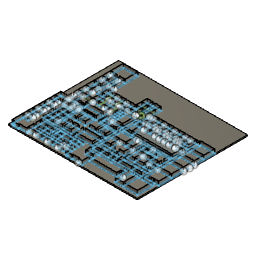
hospital_v5_v1 (Autodesk Fusion 360 design; units mm, degrees)
Autodesk Fusion 360 part; units mm, degrees
(part 1 of 2)
sketch "Sketch1" plane through (0, 0, 0) normal (0, 1, 0) x (1, 0, 0)
  line L0 (-43200, 1200) -> (-48800, 1200)
  line L1 (-48800, 1200) -> (-48800, -38423.7542)
  line L2 (-48800, -38423.7542) -> (-47000, -38423.7542)
  line L3 (-47000, -38423.7542) -> (-47000, -39400)
  line L4 (-47000, -39400) -> (-42700, -39400)
  line L5 (-42700, -39400) -> (-42700, -38500)
  line L6 (-42700, -38500) -> (-36000, -38500)
  line L7 (-36000, -38500) -> (-36000, -37042.096)
  line L8 (-43200, 900) -> (-48500, 900)
  line L9 (-48500, 900) -> (-48500, -38123.7542)
  line L10 (-48500, -38123.7542) -> (-46700, -38123.7542)
  line L11 (-46700, -38123.7542) -> (-46700, -39100)
  line L12 (-46700, -39100) -> (-43000, -39100)
  line L13 (-43000, -39100) -> (-43000, -38200)
  line L14 (-43000, -38200) -> (-36300, -38200)
  line L15 (-36300, -38200) -> (-36300, -37042.096)
  line L16 (-43200, 1200) -> (-43200, 4000)
  line L17 (-43200, 4000) -> (-42900, 4000)
  line L18 (-42900, 4000) -> (-42900, 2400)
  line L19 (-42900, 2400) -> (-39400, 2400)
  line L20 (-39400, 2400) -> (-39400, 9200)
  line L21 (-39400, 9200) -> (-42900, 9200)
  line L22 (-42900, 9200) -> (-42900, 5600)
  line L23 (-42900, 5600) -> (-43200, 5600)
  line L24 (-43200, 5600) -> (-43200, 45841.5562)
  line L25 (-43200, 45841.5562) -> (-31093.7265, 45841.5562)
  line L26 (-31093.7265, 45841.5562) -> (-31093.7265, 22000)
  line L27 (-31093.7265, 22000) -> (-9000, 22000)
  line L28 (-9000, 22000) -> (-9000, 31000)
  line L29 (-9000, 31000) -> (-4200, 31000)
  line L30 (-4200, 31000) -> (-4200, 27800)
  line L31 (-43200, 3700) -> (-43200, 2100)
  line L32 (-43200, 9500) -> (-43200, 5900)
  line L33 (-4500, 30700) -> (-4500, 27800)
  line L34 (-8700, 30700) -> (-4500, 30700)
  line L35 (-31393.7265, 21700) -> (-8700, 21700)
  line L36 (-31393.7265, 45541.5562) -> (-31393.7265, 21700)
  line L37 (-42900, 45541.5562) -> (-31393.7265, 45541.5562)
  line L38 (-42900, 9500) -> (-42900, 45541.5562)
  line L39 (-39100, 9500) -> (-42900, 9500)
  line L40 (-39100, 2100) -> (-39100, 9500)
  line L41 (-42900, 2100) -> (-39100, 2100)
  line L42 (-42900, 900) -> (-42900, 2100)
  line L43 (-42900, 900) -> (-48500, 900)
  line L44 (-48500, 900) -> (-48500, -38123.7542)
  line L45 (-48500, -38123.7542) -> (-46700, -38123.7542)
  line L46 (-46700, -38123.7542) -> (-46700, -39100)
  line L47 (-46700, -39100) -> (-43000, -39100)
  line L48 (-43000, -39100) -> (-43000, -38200)
  line L49 (-43000, -38200) -> (-36300, -38200)
  line L50 (-36300, -38200) -> (-36300, -37042.096)
  line L51 (-4200, 27800) -> (-4500, 27800)
  line L52 (-42900, 35048.3109) -> (-42900, 35074.8344)
  line L53 (-42900, 29017.6863) -> (-38000, 29017.6863)
  line L54 (-38000, 29017.6863) -> (-38000, 34000)
  line L55 (-42900, 35646.5956) -> (-37766.6149, 35646.5956)
  line L56 (-37766.6149, 35646.5956) -> (-37766.6149, 35346.5956)
  line L57 (-37766.6149, 35346.5956) -> (-42900, 35346.5956)
  line L58 (-42900, 35346.5956) -> (-42900, 35646.5956)
  line L59 (-35993.9818, 35346.5956) -> (-31393.7265, 35346.5956)
  line L60 (-31393.7265, 35346.5956) -> (-31393.7265, 35646.5956)
  line L61 (-31393.7265, 35646.5956) -> (-35993.9818, 35646.5956)
  line L62 (-35993.9818, 35646.5956) -> (-35993.9818, 35346.5956)
  line L63 (-42900, 28717.6863) -> (-37700, 28717.6863)
  line L64 (-37700, 28717.6863) -> (-37700, 34000)
  line L65 (-38000, 34000) -> (-37700, 34000)
  line L66 (-37700, 28717.6863) -> (-37700, 23500)
  line L67 (-37700, 23500) -> (-38000, 23500)
  line L68 (-38000, 23500) -> (-38000, 28717.6863)
  line L69 (-38000, 22500) -> (-42900, 22500)
  line L70 (-42900, 22500) -> (-42900, 22200)
  line L71 (-42900, 22200) -> (-38000, 22200)
  line L72 (-38000, 22200) -> (-38000, 22500)
  line L73 (-42900, 15894.4389) -> (-38184.1215, 15894.4389)
  line L74 (-38184.1215, 15894.4389) -> (-38184.1215, 21000)
  line L75 (-38184.1215, 21000) -> (-37884.1215, 21000)
  line L76 (-37884.1215, 21000) -> (-37884.1215, 10500)
  line L77 (-37884.1215, 15594.4389) -> (-37884.1215, 20700)
  line L78 (-42900, 15594.4389) -> (-38184.1215, 15594.4389)
  line L79 (-38184.1215, 15594.4389) -> (-38184.1215, 10500)
  line L80 (-38184.1215, 10500) -> (-37884.1215, 10500)
  line L81 (-31393.7265, 26975.7665) -> (-35176.305, 26975.7665)
  line L82 (-35176.305, 26975.7665) -> (-35176.305, 34204.0089)
  line L83 (-35176.305, 34204.0089) -> (-35476.305, 34204.0089)
  line L84 (-35476.305, 34204.0089) -> (-35476.305, 18232.4873)
  line L85 (-35476.305, 18232.4873) -> (-35176.305, 18232.4873)
  line L86 (-35476.305, 26675.7665) -> (-35476.305, 33904.0089)
  line L87 (-31393.7265, 26675.7665) -> (-35176.305, 26675.7665)
  line L88 (-35176.305, 26675.7665) -> (-35176.305, 18532.4873)
  line L89 (-35176.305, 18232.4873) -> (-35176.305, 18532.4873)
  line L90 (-31393.7265, 21700) -> (-31393.7265, 17176.0979)
  line L91 (-31393.7265, 17176.0979) -> (-35500, 17176.0979)
  line L92 (-35500, 17176.0979) -> (-35500, 16876.0979)
  line L93 (-35500, 16876.0979) -> (-29216.2, 16876.0979)
  line L94 (-29216.2, 16876.0979) -> (-29216.2, 17026.0979)
  line L95 (-29216.2, 17026.0979) -> (-29216.2, 17176.0979)
  line L96 (-29216.2, 17176.0979) -> (-31100, 17176.0979)
  line L97 (-31100, 17176.0979) -> (-31100, 21700)
  line L98 (-27716.2, 16974.86) -> (-28016.2, 16974.86)
  line L99 (-28016.2, 16974.86) -> (-28016.2, 21700)
  line L100 (-28016.2, 21700) -> (-27716.2, 21700)
  line L101 (-27716.2, 21700) -> (-27716.2, 16974.86)
  line L102 (-24100, 21700) -> (-24100, 17200)
  line L103 (-24100, 17200) -> (-26516.2, 17200)
  line L104 (-26516.2, 17200) -> (-26516.2, 16900)
  line L105 (-26516.2, 16900) -> (-21500, 16900)
  line L106 (-23800, 16900) -> (-26216.2, 16900)
  line L107 (-23800, 21700) -> (-23800, 17200)
  line L108 (-23800, 17200) -> (-21500, 17200)
  line L109 (-21500, 16900) -> (-21500, 17200)
  line L110 (-20100, 16900) -> (-20400, 16900)
  line L111 (-20400, 16900) -> (-20400, 21700)
  line L112 (-20400, 21700) -> (-20100, 21700)
  line L113 (-20100, 21700) -> (-20100, 16900)
  line L114 (-16700, 21700) -> (-16700, 17300)
  line L115 (-16700, 17300) -> (-18900, 17300)
  line L116 (-18900, 17300) -> (-18900, 17000)
  line L117 (-18900, 17000) -> (-14100, 17000)
  line L118 (-16400, 17000) -> (-18600, 17000)
  line L119 (-16400, 21700) -> (-16400, 17300)
  line L120 (-16400, 17300) -> (-14100, 17300)
  line L121 (-14100, 17300) -> (-14100, 17000)
  line L122 (-13000, 17000) -> (-12700, 17000)
  line L123 (-12700, 17000) -> (-12700, 21700)
  line L124 (-12700, 21700) -> (-13000, 21700)
  line L125 (-13000, 21700) -> (-13000, 17000)
  line L126 (-8700, 21700) -> (-8700, 17200)
  line L127 (-8700, 17200) -> (-11200, 17200)
  line L128 (-11200, 17200) -> (-11200, 16900)
  line L129 (-11200, 16900) -> (-4300, 16900)
  line L130 (-4300, 16900) -> (-4300, 17200)
  line L131 (-4300, 17200) -> (-8400, 17200)
  line L132 (-4600, 16900) -> (-8400, 16900)
  line L133 (-8400, 16900) -> (-10900, 16900)
  line L134 (-8400, 21700) -> (-8400, 17200)
  line L135 (-8400, 17200) -> (-4600, 17200)
  line L136 (-8400, 21700) -> (-8400, 21900)
  line L137 (-8400, 21900) -> (-4500, 21900)
  line L138 (-4500, 21900) -> (-4500, 18400)
  line L139 (-4500, 18400) -> (-4200, 18400)
  line L140 (-4200, 18400) -> (-4200, 22200)
  line L141 (-4200, 22200) -> (-8684.9202, 22200)
  line L142 (-8684.9202, 22200) -> (-8684.9202, 26300)
  line L143 (-8684.9202, 26300) -> (-4500, 26300)
  line L144 (-4500, 26300) -> (-4500, 23100)
  line L145 (-4500, 23100) -> (-4200, 23100)
  line L146 (-4200, 23100) -> (-4200, 26600)
  line L147 (-4200, 26600) -> (-8400, 26600)
  line L148 (-8700, 30700) -> (-8700, 26600)
  line L149 (-8700, 26600) -> (-8400, 26600)
  line L150 (-2627.1706, 27699.3854) -> (-2627.1706, 30999.3854)
  line L151 (-2627.1706, 30999.3854) -> (2372.8294, 30999.3854)
  line L152 (2372.8294, 30999.3854) -> (2372.8294, 22038.2459)
  line L153 (2372.8294, 22038.2459) -> (42278.3615, 22038.2459)
  line L154 (42278.3615, 22038.2459) -> (42278.3615, 22999.3854)
  line L155 (42278.3615, 22999.3854) -> (53772.8294, 22999.3854)
  line L156 (53772.8294, 22999.3854) -> (53772.8294, 2299.3854)
  line L157 (-2327.1706, 27699.3854) -> (-2327.1706, 30699.3854)
  line L158 (-2327.1706, 30699.3854) -> (2072.8294, 30699.3854)
  line L159 (2072.8294, 30699.3854) -> (2072.8294, 21738.2459)
  line L160 (2072.8294, 21738.2459) -> (42578.3615, 21738.2459)
  line L161 (42578.3615, 21738.2459) -> (42578.3615, 22699.3854)
  line L162 (42578.3615, 22699.3854) -> (53472.8294, 22699.3854)
  line L163 (53472.8294, 22699.3854) -> (53472.8294, 2299.3854)
  line L164 (-2627.1706, 27699.3854) -> (-2327.1706, 27699.3854)
  line L165 (-2600, 22900) -> (-2600, 26500)
  line L166 (-2600, 26500) -> (2072.8294, 26500)
  line L167 (-2600, 22900) -> (-2300, 22900)
  line L168 (-2300, 22900) -> (-2300, 26200)
  line L169 (-2300, 26200) -> (2072.8294, 26200)
  line L170 (-2400, 22200) -> (2072.8294, 22200)
  line L171 (2072.8294, 22200) -> (2072.8294, 21900)
  line L172 (2072.8294, 21900) -> (-2400, 21900)
  line L173 (-2400, 21900) -> (-2400, 22200)
  line L174 (1800, 21900) -> (1800, 19900)
  line L175 (1800, 19900) -> (4200, 19900)
  line L176 (2100, 21900) -> (2100, 20200)
  line L177 (2100, 20200) -> (4200, 20200)
  line L178 (4200, 19900) -> (4200, 20200)
  line L179 (2100, 19500) -> (2100, 17000)
  line L180 (2100, 17000) -> (-2200, 17000)
  line L181 (-2200, 17000) -> (-2200, 19500)
  line L182 (1400, 19500) -> (1400, 17700)
  line L183 (1400, 17700) -> (-1300, 17700)
  line L184 (-1300, 17700) -> (-1300, 19500)
  line L185 (-2200, 19500) -> (-1300, 19500)
  line L186 (1400, 19500) -> (2100, 19500)
  line L187 (5059.5443, 21738.2459) -> (5059.5443, 17199.3854)
  line L188 (5059.5443, 17199.3854) -> (8300, 17199.3854)
  line L189 (5359.5443, 21738.2459) -> (5359.5443, 17499.3854)
  line L190 (5359.5443, 17499.3854) -> (8300, 17499.3854)
  line L191 (8300, 17199.3854) -> (8300, 17499.3854)
  line L192 (9400, 17200) -> (9700, 17200)
  line L193 (9700, 17200) -> (9700, 21738.2459)
  line L194 (9700, 21738.2459) -> (9400, 21738.2459)
  line L195 (9400, 21738.2459) -> (9400, 17200)
  line L196 (13696.8067, 21738.2459) -> (13696.8067, 17599.3854)
  line L197 (13696.8067, 17599.3854) -> (10700, 17599.3854)
  line L198 (10700, 17599.3854) -> (10700, 17299.3854)
  line L199 (10700, 17299.3854) -> (16618.3238, 17299.3854)
  line L200 (13996.8067, 17299.3854) -> (11000, 17299.3854)
  line L201 (13996.8067, 21738.2459) -> (13996.8067, 17599.3854)
  line L202 (13996.8067, 17599.3854) -> (16618.3238, 17599.3854)
  line L203 (16618.3238, 17299.3854) -> (16618.3238, 17599.3854)
  line L204 (18000, 17400) -> (18300, 17400)
  line L205 (18300, 17400) -> (18300, 21738.2459)
  line L206 (18300, 21738.2459) -> (18000, 21738.2459)
  line L207 (18000, 21738.2459) -> (18000, 17400)
  line L208 (22221.7642, 21738.2459) -> (22221.7642, 17599.3854)
  line L209 (22221.7642, 17599.3854) -> (19200, 17599.3854)
  line L210 (19200, 17599.3854) -> (19200, 17299.3854)
  line L211 (19200, 17299.3854) -> (25200, 17299.3854)
  line L212 (22521.7642, 17299.3854) -> (19500, 17299.3854)
  line L213 (22521.7642, 21738.2459) -> (22521.7642, 17599.3854)
  line L214 (22521.7642, 17599.3854) -> (25200, 17599.3854)
  line L215 (25200, 17299.3854) -> (25200, 17599.3854)
  line L216 (26000, 17300) -> (26300, 17300)
  line L217 (26300, 17300) -> (26300, 21917.4863)
  line L218 (26300, 21917.4863) -> (26000, 21917.4863)
  line L219 (26000, 21917.4863) -> (26000, 17300)
  line L220 (30675.2551, 21738.2459) -> (30675.2551, 17599.3854)
  line L221 (30675.2551, 17599.3854) -> (27700, 17599.3854)
  line L222 (27700, 17599.3854) -> (27700, 17299.3854)
  line L223 (27700, 17299.3854) -> (33500, 17299.3854)
  line L224 (30975.2551, 17299.3854) -> (28000, 17299.3854)
  line L225 (30975.2551, 21738.2459) -> (30975.2551, 17599.3854)
  line L226 (30975.2551, 17599.3854) -> (33500, 17599.3854)
  line L227 (33500, 17599.3854) -> (33500, 17299.3854)
  line L228 (37400, 16899.3854) -> (34800, 16899.3854)
  line L229 (34800, 16899.3854) -> (34800, 21738.2459)
  line L230 (37400, 17199.3854) -> (35100, 17199.3854)
  line L231 (35100, 17199.3854) -> (35100, 21738.2459)
  line L232 (37400, 16899.3854) -> (37400, 17199.3854)
  line L233 (39957.4234, 21738.2459) -> (40257.4234, 21738.2459)
  line L234 (40257.4234, 21738.2459) -> (40257.4234, -4527.77)
  line L235 (40257.4234, -4527.77) -> (39957.4234, -4527.77)
  line L236 (39957.4234, -4527.77) -> (39957.4234, 21738.2459)
  line L237 (39957.4234, 14808.2859) -> (35895.4106, 14808.2859)
  line L238 (35895.4106, 14808.2859) -> (35895.4106, 14508.2859)
  line L239 (35895.4106, 14508.2859) -> (39957.4234, 14508.2859)
  line L240 (39957.4234, 14508.2859) -> (39957.4234, 14808.2859)
  line L241 (34800, 14800) -> (34800, 10500)
  line L242 (34800, 10500) -> (39957.4234, 10500)
  line L243 (34500, 14800) -> (34500, 10200)
  line L244 (34500, 10200) -> (39957.4234, 10200)
  line L245 (34500, 14800) -> (34800, 14800)
  line L246 (27100, 14800) -> (33200, 14800)
  line L247 (33200, 14800) -> (33200, 14500)
  line L248 (33200, 14500) -> (30044.2434, 14500)
  line L249 (30044.2434, 14500) -> (30044.2434, 10500)
  line L250 (30044.2434, 10500) -> (34500, 10500)
  line L251 (32900, 14800) -> (29744.2434, 14800)
  line L252 (27100, 14500) -> (29744.2434, 14500)
  line L253 (29744.2434, 14500) -> (29744.2434, 10200)
  line L254 (29744.2434, 10200) -> (34500, 10200)
  line L255 (26188.0475, 14800) -> (26188.0475, 10505.8366)
  line L256 (26188.0475, 10505.8366) -> (29744.2434, 10505.8366)
  line L257 (27100, 14800) -> (27100, 14500)
  line L258 (25888.0475, 14800) -> (25888.0475, 10205.8366)
  line L259 (25888.0475, 10205.8366) -> (29744.2434, 10205.8366)
  line L260 (25888.0475, 14800) -> (26188.0475, 14800)
  line L261 (19100, 14900) -> (25100, 14900)
  line L262 (25100, 14900) -> (25100, 14600)
  line L263 (25100, 14600) -> (22123.4454, 14600)
  line L264 (22123.4454, 14600) -> (22123.4454, 10516.3322)
  line L265 (22123.4454, 10516.3322) -> (25888.0475, 10516.3322)
  line L266 (24800, 14900) -> (21823.4454, 14900)
  line L267 (19100, 14600) -> (21823.4454, 14600)
  line L268 (21823.4454, 14600) -> (21823.4454, 10216.3322)
  line L269 (21823.4454, 10216.3322) -> (25888.0475, 10216.3322)
  line L270 (19100, 14600) -> (19100, 14900)
  line L271 (18400, 14873.3559) -> (18400, 10518.6501)
  line L272 (18400, 10518.6501) -> (21823.4454, 10518.6501)
  line L273 (18100, 14873.3559) -> (18100, 10218.6501)
  line L274 (18100, 10218.6501) -> (21823.4454, 10218.6501)
  line L275 (18100, 14873.3559) -> (18400, 14873.3559)
  line L276 (10486.8954, 15164.2595) -> (16492.6493, 15164.2595)
  line L277 (16492.6493, 15164.2595) -> (16492.6493, 14864.2595)
  line L278 (16492.6493, 14864.2595) -> (13938.1571, 14864.2595)
  line L279 (13938.1571, 14864.2595) -> (13938.1571, 10518.6501)
  line L280 (13938.1571, 10518.6501) -> (18100, 10518.6501)
  line L281 (16192.6493, 15164.2595) -> (13638.1571, 15164.2595)
  line L282 (10486.8954, 14864.2595) -> (13638.1571, 14864.2595)
  line L283 (13638.1571, 14864.2595) -> (13638.1571, 10218.6501)
  line L284 (13638.1571, 10218.6501) -> (18100, 10218.6501)
  line L285 (10486.8954, 14864.2595) -> (10486.8954, 15164.2595)
  line L286 (9184.0997, 15032.9096) -> (9484.0997, 15032.9096)
  line L287 (9484.0997, 15032.9096) -> (9484.0997, 10518.6501)
  line L288 (9484.0997, 10518.6501) -> (13638.1571, 10518.6501)
  line L289 (9184.0997, 14732.9096) -> (9184.0997, 10218.6501)
  line L290 (9184.0997, 10218.6501) -> (13638.1571, 10218.6501)
  line L291 (9184.0997, 14732.9096) -> (9184.0997, 15032.9096)
  line L292 (9184.0997, 10518.6501) -> (5300, 10518.6501)
  line L293 (5300, 10518.6501) -> (5300, 14900)
  line L294 (5300, 14900) -> (8300, 14900)
  line L295 (8300, 15200) -> (2300, 15200)
  line L296 (8300, 14900) -> (8300, 15200)
  line L297 (5000, 15200) -> (8000, 15200)
  line L298 (9184.0997, 10218.6501) -> (5000, 10218.6501)
  line L299 (5000, 10218.6501) -> (5000, 14900)
  line L300 (5000, 14900) -> (2300, 14900)
  line L301 (2300, 15200) -> (2300, 14900)
  line L302 (1200, 15050) -> (1200, 10518.6501)
  line L303 (1200, 10518.6501) -> (5000, 10518.6501)
  line L304 (1200, 15050) -> (900, 15050)
  line L305 (900, 15050) -> (900, -2285.7896)
  line L306 (900, -2285.7896) -> (1200, -2285.7896)
  line L307 (1200, -2285.7896) -> (1200, 15050)
  line L308 (5000, 10218.6501) -> (1200, 10218.6501)
  line L309 (1200, 2183.5992) -> (39957.4234, 2183.5992)
  line L310 (39957.4234, 2183.5992) -> (39957.4234, 1883.5992)
  line L311 (39957.4234, 1883.5992) -> (1200, 1883.5992)
  line L312 (1200, 1883.5992) -> (1200, 2183.5992)
  line L313 (7687.3645, 2183.5992) -> (7387.3645, 2183.5992)
  line L314 (7387.3645, 2183.5992) -> (7387.3645, 10218.6501)
  line L315 (7387.3645, 10218.6501) -> (7687.3645, 10218.6501)
  line L316 (7687.3645, 10218.6501) -> (7687.3645, 2183.5992)
  line L317 (900, -3456.7838) -> (1200, -3456.7838)
  line L318 (1200, -3456.7838) -> (1200, -21629.9336)
  line L319 (1200, -21629.9336) -> (900, -21629.9336)
  line L320 (900, -21629.9336) -> (900, -3456.7838)
  line L321 (1200, 400) -> (8272.1931, 400)
  line L322 (8272.1931, 400) -> (8272.1931, 100)
  line L323 (8272.1931, 100) -> (1200, 100)
  line L324 (1200, 100) -> (1200, 400)
  line L325 (9600, 400) -> (15300, 400)
  line L326 (15300, 100) -> (15300, 400)
  line L327 (15300, 100) -> (13100, 100)
  line L328 (13100, 100) -> (13100, -8100)
  line L329 (13100, -8100) -> (18600, -8100)
  line L330 (18600, -8100) -> (18600, 100)
  line L331 (18600, 100) -> (16675.3959, 100)
  line L332 (15000, 400) -> (12800, 400)
  line L333 (9600, 100) -> (12800, 100)
  line L334 (12800, 100) -> (12800, -8400)
  line L335 (12800, -8400) -> (18900, -8400)
  line L336 (18900, -8400) -> (18900, 400)
  line L337 (18900, 400) -> (16675.3959, 400)
  line L338 (9600, 400) -> (9600, 100)
  line L339 (16675.3959, 400) -> (16675.3959, 100)
  line L340 (12800, -8100) -> (1200, -8100)
  line L341 (1200, -8100) -> (1200, -8400)
  line L342 (1200, -8400) -> (12800, -8400)
  line L343 (12800, -8400) -> (12800, -8100)
  line L344 (21000, 500) -> (28000, 500)
  line L345 (28000, 500) -> (28000, 200)
  line L346 (21000, 500) -> (21000, -2283.3657)
  line L347 (21300, 200) -> (27700, 200)
  line L348 (21300, 200) -> (21300, -2283.3657)
  line L349 (27700, 200) -> (28000, 200)
  line L350 (21300, -2283.3657) -> (21000, -2283.3657)
  line L351 (21275.4064, -3692.4683) -> (26198.4602, -3692.4683)
  line L352 (26198.4602, -3692.4683) -> (26198.4602, 200)
  line L353 (21275.4064, -3992.4683) -> (26498.4602, -3992.4683)
  line L354 (26498.4602, -3992.4683) -> (26498.4602, 200)
  line L355 (21275.4064, -3992.4683) -> (21275.4064, -3692.4683)
  line L356 (29042.4636, 331.8561) -> (29042.4636, -3200)
  line L357 (29042.4636, -3200) -> (26498.4602, -3200)
  line L358 (29342.4636, 331.8561) -> (29342.4636, -3500)
  line L359 (29342.4636, -3500) -> (26498.4602, -3500)
  line L360 (29042.4636, 331.8561) -> (29342.4636, 331.8561)
  line L361 (30100, 600) -> (39405.6299, 600)
  line L362 (39405.6299, 600) -> (39405.6299, 300)
  line L363 (39405.6299, 300) -> (30100, 300)
  line L364 (30100, 300) -> (30100, 600)
  line L365 (39405.6299, 600) -> (39957.4234, 600)
  line L366 (39405.6299, 300) -> (39957.4234, 300)
  line L367 (26498.4602, -3500) -> (32700, -3500)
  line L368 (32700, -3500) -> (32700, -8200)
  line L369 (32700, -8200) -> (26498.4602, -8200)
  line L370 (26498.4602, -8200) -> (26498.4602, -3500)
  line L371 (26198.4602, -3200) -> (33000, -3200)
  line L372 (33000, -3200) -> (33000, -8500)
  line L373 (33000, -8500) -> (26198.4602, -8500)
  line L374 (26198.4602, -8500) -> (26198.4602, -3200)
  line L375 (32700, -3200) -> (32700, 300)
  line L376 (33000, -3200) -> (33000, 300)
  line L377 (33000, -8200) -> (39478.3598, -8200)
  line L378 (39957.4234, -8200) -> (39478.3598, -8200)
  line L379 (39957.4234, -8200) -> (39957.4234, -6500)
  line L380 (40257.4234, -6500) -> (40257.4234, -8500)
  line L381 (40257.4234, -8500) -> (33000, -8500)
  line L382 (39957.4234, -6500) -> (40257.4234, -6500)
  line L383 (26198.4602, -8200) -> (21500, -8200)
  line L384 (21500, -8200) -> (21500, -5500)
  line L385 (26198.4602, -8500) -> (21200, -8500)
  line L386 (21200, -8500) -> (21200, -5500)
  line L387 (21500, -5500) -> (21200, -5500)
  line L388 (21500, -9500) -> (21500, -8500)
  line L389 (21500, -9500) -> (21200, -9500)
  line L390 (21200, -9500) -> (21200, -8500)
  line L391 (40257.4234, -8500) -> (39957.4234, -8500)
  line L392 (39957.4234, -8500) -> (39957.4234, -15700.4213)
  line L393 (39957.4234, -15700.4213) -> (40257.4234, -15700.4213)
  line L394 (40257.4234, -15700.4213) -> (40257.4234, -8500)
  line L395 (39957.4234, -11251.2465) -> (36984.7278, -11251.2465)
  line L396 (36984.7278, -11251.2465) -> (36984.7278, -11551.2465)
  line L397 (36984.7278, -11551.2465) -> (39957.4234, -11551.2465)
  line L398 (39957.4234, -11551.2465) -> (39957.4234, -11251.2465)
  line L399 (36055.0377, -11251.2465) -> (34969.0281, -11251.2465)
  line L400 (34969.0281, -11251.2465) -> (34969.0281, -11551.2465)
  line L401 (34969.0281, -11551.2465) -> (36055.0377, -11551.2465)
  line L402 (36055.0377, -11551.2465) -> (36055.0377, -11251.2465)
  line L403 (34969.0281, -8500) -> (34969.0281, -11251.2465)
  line L404 (34969.0281, -11551.2465) -> (34969.0281, -15500)
  line L405 (34969.0281, -15500) -> (37000, -15500)
  line L406 (34669.0281, -11551.2465) -> (34669.0281, -15800)
  line L407 (34669.0281, -15800) -> (37000, -15800)
  line L408 (34669.0281, -11551.2465) -> (34669.0281, -8500)
  line L409 (37000, -15800) -> (37000, -15500)
  line L410 (39957.4234, -15700.4213) -> (38700, -15700.4213)
  line L411 (38700, -15700.4213) -> (38700, -15400)
  line L412 (38700, -15400) -> (39957.4234, -15400)
  line L413 (39957.4234, -15400) -> (39957.4234, -15700.4213)
  line L414 (21542.5002, -10826.841) -> (21542.5002, -15500)
  line L415 (21542.5002, -15500) -> (27200.1552, -15500)
  line L416 (27200.1552, -15500) -> (27200.1552, -8500)
  line L417 (21242.5002, -10826.841) -> (21242.5002, -15800)
  line L418 (21242.5002, -15800) -> (27500.1552, -15800)
  line L419 (27500.1552, -15800) -> (27500.1552, -8500)
  line L420 (21242.5002, -10826.841) -> (21542.5002, -10826.841)
  line L421 (27500.1552, -15800) -> (34669.0281, -15800)
  line L422 (34669.0281, -15800) -> (34669.0281, -15500)
  line L423 (34669.0281, -15500) -> (27500.1552, -15500)
  line L424 (27500.1552, -15500) -> (27500.1552, -15800)
  line L425 (40500, -18091.598) -> (40500, -23000)
  line L426 (40500, -23000) -> (21247.3182, -23000)
  line L427 (21247.3182, -23000) -> (21247.3182, -18091.598)
  line L428 (40200, -22700) -> (21547.3182, -22700)
  line L429 (21547.3182, -22700) -> (21547.3182, -18391.598)
  line L430 (40200, -18391.598) -> (40200, -22700)
  line L431 (23477.5822, -18091.598) -> (23477.5822, -18391.598)
  line L432 (22428.0462, -18391.598) -> (22428.0462, -18091.598)
  line L433 (32021.4612, -18391.598) -> (32321.4612, -18391.598)
  line L434 (32321.4612, -18391.598) -> (32321.4612, -22700)
  line L435 (32321.4612, -22700) -> (32021.4612, -22700)
  line L436 (32021.4612, -22700) -> (32021.4612, -18391.598)
  line L437 (37515.1262, -18091.598) -> (37515.1262, -18391.598)
  line L438 (36022.8172, -18391.598) -> (36022.8172, -18091.598)
  line L439 (21547.3182, -18391.598) -> (22428.0462, -18391.598)
  line L440 (21247.3182, -18091.598) -> (22428.0462, -18091.598)
  line L441 (23477.5822, -18091.598) -> (36022.8172, -18091.598)
  line L442 (37515.1262, -18091.598) -> (40500, -18091.598)
  line L443 (23477.5822, -18391.598) -> (36022.8172, -18391.598)
  line L444 (37515.1262, -18391.598) -> (40200, -18391.598)
  line L445 (4000, -15500) -> (1200, -15500)
  line L446 (1200, -15500) -> (1200, -15800)
  line L447 (1200, -15800) -> (4000, -15800)
  line L448 (4000, -15800) -> (4000, -15500)
  line L449 (5300, -15500) -> (7800, -15500)
  line L450 (7800, -15500) -> (7800, -8400)
  line L451 (5300, -15800) -> (8100, -15800)
  line L452 (8100, -15800) -> (8100, -8400)
  line L453 (5300, -15800) -> (5300, -15500)
  line L454 (8100, -15800) -> (11800, -15800)
  line L455 (11800, -15800) -> (11800, -15500)
  line L456 (11800, -15500) -> (8100, -15500)
  line L457 (18600, -8400) -> (18600, -15400)
  line L458 (18600, -15400) -> (15000, -15400)
  line L459 (18900, -8400) -> (18900, -15700)
  line L460 (18900, -15700) -> (15000, -15700)
  line L461 (15000, -15700) -> (15000, -15400)
  line L462 (1200, -18044.864) -> (11761.3443, -18044.864)
  line L463 (11761.3443, -18344.864) -> (1200, -18344.864)
  line L464 (11761.3443, -18044.864) -> (11761.3443, -18344.864)
  line L465 (15034.8266, -18199.5167) -> (17500, -18199.5167)
  line L466 (17500, -18199.5167) -> (17500, -23000)
  line L467 (15034.8266, -18499.5167) -> (17200, -18499.5167)
  line L468 (17200, -18499.5167) -> (17200, -23000)
  line L469 (17200, -23000) -> (13797.6049, -23000)
  line L470 (13797.6049, -23000) -> (13797.6049, -18276.8431)
  line L471 (13797.6049, -18276.8431) -> (13497.6049, -18276.8431)
  line L472 (13497.6049, -18276.8431) -> (13497.6049, -23000)
  line L473 (13497.6049, -23000) -> (7500, -23000)
  line L474 (17500, -23000) -> (19500, -23000)
  line L475 (19500, -23000) -> (19500, -23300)
  line L476 (19500, -23300) -> (900, -23300)
  line L477 (900, -23300) -> (900, -22194.7116)
  line L478 (1200, -22194.7116) -> (1200, -23000)
  line L479 (1200, -23000) -> (7500, -23000)
  line L480 (900, -22194.7116) -> (1200, -22194.7116)
  line L481 (7379.5177, -18344.864) -> (7679.5177, -18344.864)
  line L482 (7679.5177, -18344.864) -> (7679.5177, -23000)
  line L483 (7679.5177, -23000) -> (7379.5177, -23000)
  line L484 (7379.5177, -23000) -> (7379.5177, -18344.864)
  line L485 (53472.8294, 2299.3854) -> (53772.8294, 2299.3854)
  line L486 (53772.8294, 2299.3854) -> (53772.8294, -22534.0367)
  line L487 (53772.8294, -22534.0367) -> (53472.8294, -22534.0367)
  line L488 (53472.8294, -22534.0367) -> (53472.8294, 2299.3854)
  line L489 (42578.3615, 21738.2459) -> (42278.3615, 21738.2459)
  line L490 (42278.3615, 21738.2459) -> (42278.3615, 12416.3292)
  line L491 (42278.3615, 12416.3292) -> (42578.3615, 12416.3292)
  line L492 (42578.3615, 12416.3292) -> (42578.3615, 21738.2459)
  line L493 (42578.3615, 14197.2396) -> (53472.8294, 14197.2396)
  line L494 (53472.8294, 14197.2396) -> (53472.8294, 13897.2396)
  line L495 (53472.8294, 13897.2396) -> (42578.3615, 13897.2396)
  line L496 (42578.3615, 13897.2396) -> (42578.3615, 14197.2396)
  line L497 (42600, 10000) -> (42600, 6600)
  line L498 (42600, 6600) -> (53472.8294, 6600)
  line L499 (42300, 10000) -> (42300, 6300)
  line L500 (42300, 6300) -> (53472.8294, 6300)
  line L501 (42300, 6300) -> (42600, 6300)
  line L502 (42600, 6300) -> (42600, 5600)
  line L503 (42600, 5600) -> (42300, 5600)
  line L504 (42300, 5600) -> (42300, 6300)
  line L505 (42300, 10000) -> (42600, 10000)
  line L506 (42600, 4300) -> (42600, -2000)
  line L507 (42600, -2000) -> (53472.8294, -2000)
  line L508 (42300, 4300) -> (42300, -2300)
  line L509 (42300, -2300) -> (53472.8294, -2300)
  line L510 (42300, 4300) -> (42600, 4300)
  line L511 (42600, -2300) -> (42300, -2300)
  line L512 (42300, -2300) -> (42300, -6400)
  line L513 (42300, -6400) -> (42600, -6400)
  line L514 (42600, -6400) -> (42600, -2300)
  line L515 (42300, -7900) -> (42600, -7900)
  line L516 (42600, -7900) -> (42600, -12000)
  line L517 (42600, -12000) -> (42300, -12000)
  line L518 (42300, -12000) -> (42300, -7900)
  line L519 (42600, -12000) -> (53472.8294, -12000)
  line L520 (53472.8294, -12000) -> (53472.8294, -11700)
  line L521 (53472.8294, -11700) -> (42600, -11700)
  line L522 (42600, -11700) -> (42600, -12000)
  line L523 (42300, -12000) -> (42300, -22500)
  line L524 (42300, -22500) -> (46500, -22500)
  line L525 (42600, -12000) -> (42600, -22200)
  line L526 (42600, -22200) -> (46500, -22200)
  line L527 (46500, -22200) -> (46500, -22500)
  line L528 (47677.7349, -22500) -> (47677.7349, -22200)
  line L529 (47677.7349, -22200) -> (53472.8294, -22200)
  line L530 (47677.7349, -22500) -> (53472.8294, -22534.0367)
  line L531 (50513.1999, -23154.4586) -> (50213.1999, -23154.4586)
  line L532 (50213.1999, -23154.4586) -> (50213.1999, -22514.8917)
  line L533 (50213.1999, -22514.8917) -> (50513.1999, -22514.8917)
  line L534 (50513.1999, -22514.8917) -> (50513.1999, -23154.4586)
  line L535 (33671.9139, -24633.7608) -> (33671.9139, -37524.8224)
  line L536 (33671.9139, -37524.8224) -> (51586.1004, -37524.8224)
  line L537 (51586.1004, -37524.8224) -> (51586.1004, -24633.7608)
  line L538 (33971.9139, -37224.8224) -> (51286.1004, -37224.8224)
  line L539 (51286.1004, -37224.8224) -> (51286.1004, -24933.7608)
  line L540 (33971.9139, -24933.7608) -> (33971.9139, -37224.8224)
  line L541 (37524.6019, -24633.7608) -> (37524.6019, -24933.7608)
  line L542 (35866.483, -24933.7608) -> (35866.483, -24633.7608)
  line L543 (42629.0071, -24633.7608) -> (42629.0071, -24933.7608)
  line L544 (44043.285, -24933.7608) -> (44043.285, -24633.7608)
  line L545 (35866.483, -24933.7608) -> (33971.9139, -24933.7608)
  line L546 (35866.483, -24633.7608) -> (33671.9139, -24633.7608)
  line L547 (51286.1004, -24933.7608) -> (44043.285, -24933.7608)
  line L548 (42629.0071, -24933.7608) -> (37524.6019, -24933.7608)
  line L549 (51586.1004, -24633.7608) -> (44043.285, -24633.7608)
  line L550 (42629.0071, -24633.7608) -> (37524.6019, -24633.7608)
  line L551 (39800.4514, -24933.7608) -> (40100.4514, -24933.7608)
  line L552 (40100.4514, -24933.7608) -> (40100.4514, -37224.8224)
  line L553 (40100.4514, -37224.8224) -> (39800.4514, -37224.8224)
  line L554 (39800.4514, -37224.8224) -> (39800.4514, -24933.7608)
  line L555 (33671.9139, -31623.8698) -> (30810.846, -31623.8698)
  line L556 (30810.846, -31623.8698) -> (30810.846, -33314.5009)
  line L557 (30810.846, -33314.5009) -> (8500, -33314.5009)
  line L558 (8500, -33314.5009) -> (8500, -39000)
  line L559 (8500, -39000) -> (5207.5394, -39000)
  line L560 (33671.9139, -31323.8698) -> (30510.846, -31323.8698)
  line L561 (30510.846, -31323.8698) -> (30510.846, -33014.5009)
  line L562 (30510.846, -33014.5009) -> (8200, -33014.5009)
  line L563 (8200, -33014.5009) -> (8200, -38700)
  line L564 (8200, -38700) -> (5207.5394, -38700)
  line L565 (5207.5394, -39000) -> (5207.5394, -38700)
  line L566 (5207.5394, -38700) -> (5207.5394, -38158.809)
  line L567 (5207.5394, -38158.809) -> (330.7192, -38158.809)
  line L568 (330.7192, -38158.809) -> (330.7192, -39000)
  line L569 (330.7192, -39000) -> (-4000, -39000)
  line L570 (-4000, -39000) -> (-4000, -38158.809)
  line L571 (-4000, -38158.809) -> (-5800, -38158.809)
  line L572 (-5800, -38158.809) -> (-5800, -33352.468)
  line L573 (5507.5394, -38700) -> (5507.5394, -37858.809)
  line L574 (5507.5394, -37858.809) -> (30.7192, -37858.809)
  line L575 (30.7192, -37858.809) -> (30.7192, -38700)
  line L576 (30.7192, -38700) -> (-3700, -38700)
  line L577 (-3700, -38700) -> (-3700, -37858.809)
  line L578 (-3700, -37858.809) -> (-5500, -37858.809)
  line L579 (-5500, -37858.809) -> (-5500, -33352.468)
  line L580 (-5800, -33352.468) -> (-8600, -33352.468)
  line L581 (-8600, -33352.468) -> (-8600, -37000)
  line L582 (-5500, -33352.468) -> (-5500, -33052.468)
  line L583 (-5500, -33052.468) -> (-9000, -33052.468)
  line L584 (-9000, -33052.468) -> (-9000, -36742.096)
  line L585 (-36000, -37042.096) -> (-8600, -37042.096)
  line L586 (-8600, -37042.096) -> (-8600, -37000)
  line L587 (-9000, -36742.096) -> (-37000, -36742.096)
  line L588 (-37000, -36742.096) -> (-37000, -32200)
  line L589 (-37000, -32200) -> (-37300, -32200)
  line L590 (-37300, -32200) -> (-37300, -37042.096)
  line L591 (-37300, -37042.096) -> (-36300, -37042.096)
  line L592 (-33900, -33100) -> (-31200, -33100)
  line L593 (-31200, -33100) -> (-31200, -36742.096)
  line L594 (-33900, -32800) -> (-30900, -32800)
  line L595 (-30900, -32800) -> (-30900, -36742.096)
  line L596 (-33900, -33100) -> (-33900, -32800)
  line L597 (-30900, -32800) -> (-28000, -32800)
  line L598 (-28000, -32800) -> (-28000, -33100)
  line L599 (-28000, -33100) -> (-30900, -33100)
  line L600 (-26200, -33000) -> (-25900, -33000)
  line L601 (-25900, -33000) -> (-25900, -36742.096)
  line L602 (-25900, -36742.096) -> (-26200, -36742.096)
  line L603 (-26200, -36742.096) -> (-26200, -33000)
  line L604 (-24700, -33000) -> (-22000, -33000)
  line L605 (-22000, -33000) -> (-21900, -33000)
  line L606 (-21900, -33000) -> (-21900, -36742.096)
  line L607 (-24700, -32700) -> (-22000, -32700)
  line L608 (-22000, -32700) -> (-21600, -32700)
  line L609 (-21600, -32700) -> (-21600, -36742.096)
  line L610 (-24700, -33000) -> (-24700, -32700)
  line L611 (-21600, -32700) -> (-18800, -32700)
  line L612 (-18800, -32700) -> (-18800, -33000)
  line L613 (-18800, -33000) -> (-21600, -33000)
  line L614 (-16100, -32700) -> (-10100, -32700)
  line L615 (-10100, -32700) -> (-10100, -33000)
  line L616 (-10100, -33000) -> (-13000, -33000)
  line L617 (-13000, -33000) -> (-13000, -36742.096)
  line L618 (-10400, -32700) -> (-13300, -32700)
  line L619 (-16100, -33000) -> (-13300, -33000)
  line L620 (-13300, -33000) -> (-13300, -36742.096)
  line L621 (-16100, -33000) -> (-16100, -32700)
  line L622 (-17300, -33000) -> (-17600, -33000)
  line L623 (-17600, -33000) -> (-17600, -36742.096)
  line L624 (-17600, -36742.096) -> (-17300, -36742.096)
  line L625 (-17300, -36742.096) -> (-17300, -33000)
  line L626 (2100, -25000) -> (8400, -25000)
  line L627 (8400, -25000) -> (8400, -30000)
  line L628 (8400, -30000) -> (2100, -30000)
  line L629 (2100, -30000) -> (2100, -25000)
  line L630 (8100, -29700) -> (2400, -29700)
  line L631 (2400, -29700) -> (2400, -25300)
  line L632 (2400, -25300) -> (8100, -25300)
  line L633 (8100, -25300) -> (8100, -29700)
  line L634 (8200, -33014.5009) -> (8400, -33014.5009)
  line L635 (8400, -33014.5009) -> (8400, -30000)
  line L636 (8400, -30000) -> (8200, -30000)
  line L637 (8200, -30000) -> (8200, -33014.5009)
  line L638 (8400, -25000) -> (17400, -25000)
  line L639 (17400, -25000) -> (17400, -25300)
  line L640 (17400, -25300) -> (8400, -25300)
  line L641 (8400, -25300) -> (8400, -25000)
  line L642 (18700, -25000) -> (30700, -25000)
  line L643 (30700, -25000) -> (30700, -28000)
  line L644 (18700, -25300) -> (30400, -25300)
  line L645 (30400, -25300) -> (30400, -28000)
  line L646 (30400, -28000) -> (30700, -28000)
  line L647 (18700, -25000) -> (18700, -25300)
  line L648 (30510.846, -31323.8698) -> (30810.846, -31323.8698)
  line L649 (30810.846, -31323.8698) -> (30810.846, -29400)
  line L650 (30810.846, -29400) -> (30510.846, -29400)
  line L651 (30510.846, -29400) -> (30510.846, -31323.8698)
  line L652 (-39100, 2100) -> (-31000, 2100)
  line L653 (-31000, 2100) -> (-31000, 2400)
  line L654 (-31000, 2400) -> (-39100, 2400)
  line L655 (-39100, 2400) -> (-39100, 2100)
  line L656 (-42900, 900) -> (-32129.3248, 900)
  line L657 (-32129.3248, 900) -> (-32129.3248, 1200)
  line L658 (-32129.3248, 1200) -> (-42900, 1200)
  line L659 (-42900, 1200) -> (-42900, 900)
  line L660 (-42231.7343, -3919.6167) -> (-42531.7343, -3919.6167)
  line L661 (-42531.7343, -3919.6167) -> (-42531.7343, 900)
  line L662 (-42531.7343, 900) -> (-42231.7343, 900)
  line L663 (-42231.7343, 900) -> (-42231.7343, -3919.6167)
  line L664 (-43840.5829, -3673.2165) -> (-48500, -3673.2165)
  line L665 (-48500, -3673.2165) -> (-48500, -3973.2165)
  line L666 (-48500, -3973.2165) -> (-43840.5829, -3973.2165)
  line L667 (-43840.5829, -3973.2165) -> (-43840.5829, -3673.2165)
  line L668 (-36709.4703, 900) -> (-36709.4703, -3600)
  line L669 (-36709.4703, -3600) -> (-41100, -3600)
  line L670 (-41100, -3600) -> (-41100, -3900)
  line L671 (-41100, -3900) -> (-32000, -3900)
  line L672 (-36409.4703, -3900) -> (-40800, -3900)
  line L673 (-36409.4703, 900) -> (-36409.4703, -3600)
  line L674 (-36409.4703, -3600) -> (-32000, -3600)
  line L675 (-32000, -3600) -> (-32000, -3900)
  line L676 (-32500, -3100) -> (-32200, -3100)
  line L677 (-32200, -3100) -> (-32200, 0)
  line L678 (-32200, 0) -> (-32500, 0)
  line L679 (-32500, 0) -> (-32500, -1400)
  line L680 (-32500, -1400) -> (-36409.4703, -1400)
  line L681 (-32200, -300) -> (-32200, -1700)
  line L682 (-32500, -2800) -> (-32500, -1700)
  line L683 (-32500, -1700) -> (-36409.4703, -1700)
  line L684 (-32500, -3100) -> (-32500, -2800)
  line L685 (-31000, 2100) -> (-31300, 2100)
  line L686 (-31300, 2100) -> (-31300, 1100)
  line L687 (-31300, 1100) -> (-31000, 1100)
  line L688 (-31000, 1100) -> (-31000, 2100)
  line L689 (-31100, 200) -> (-31100, -1500)
  line L690 (-31100, -1500) -> (-17500, -1500)
  line L691 (-17500, -1500) -> (-17500, 2300)
  line L692 (-31400, 200) -> (-31400, -1800)
  line L693 (-31400, -1800) -> (-17200, -1800)
  line L694 (-17200, -1800) -> (-17200, 2300)
  line L695 (-17500, 2300) -> (-17200, 2300)
  line L696 (-31100, 200) -> (-31400, 200)
  line L697 (-44800, -29500) -> (-48500, -29500)
  line L698 (-48500, -29500) -> (-48500, -29800)
  line L699 (-48500, -29800) -> (-44800, -29800)
  line L700 (-44800, -29800) -> (-44800, -29500)
  line L701 (-44500, -28800) -> (-44500, -22800)
  line L702 (-44500, -22800) -> (-44800, -22800)
  line L703 (-44800, -22800) -> (-44800, -25600)
  line L704 (-44800, -25600) -> (-48500, -25600)
  line L705 (-44500, -23100) -> (-44500, -25900)
  line L706 (-44800, -28800) -> (-44800, -25900)
  line L707 (-44800, -25900) -> (-48500, -25900)
  line L708 (-44800, -28800) -> (-44500, -28800)
  line L709 (-44700, -21400) -> (-48500, -21400)
  line L710 (-48500, -21400) -> (-48500, -21700)
  line L711 (-48500, -21700) -> (-44700, -21700)
  line L712 (-44700, -21700) -> (-44700, -21400)
  line L713 (-44500, -20000) -> (-44500, -13873.6338)
  line L714 (-44500, -13873.6338) -> (-44800, -13873.6338)
  line L715 (-44800, -13873.6338) -> (-44800, -16700)
  line L716 (-44800, -16700) -> (-48500, -16700)
  line L717 (-44500, -14173.6338) -> (-44500, -17000)
  line L718 (-44800, -20000) -> (-44800, -17000)
  line L719 (-44800, -17000) -> (-48500, -17000)
  line L720 (-44800, -20000) -> (-44500, -20000)
  line L721 (-44800, -12300) -> (-48500, -12300)
  line L722 (-48500, -12300) -> (-48500, -12600)
  line L723 (-48500, -12600) -> (-44800, -12600)
  line L724 (-44800, -12600) -> (-44800, -12300)
  line L725 (-44500, -11200) -> (-44500, -5200)
  line L726 (-44500, -5200) -> (-44800, -5200)
  line L727 (-44800, -5200) -> (-44800, -8100)
  line L728 (-44800, -8100) -> (-48500, -8100)
  line L729 (-44500, -5500) -> (-44500, -8400)
  line L730 (-44800, -11200) -> (-44800, -8400)
  line L731 (-44800, -8400) -> (-48500, -8400)
  line L732 (-44800, -11200) -> (-44500, -11200)
  line L733 (-40325.557, -11824.224) -> (-40325.557, -5000)
  line L734 (-40325.557, -5000) -> (-32101.2083, -5000)
  line L735 (-40025.557, -11824.224) -> (-40025.557, -5300)
  line L736 (-40025.557, -5300) -> (-32101.2083, -5300)
  line L737 (-32101.2083, -5000) -> (-32101.2083, -5300)
  line L738 (-40025.557, -11824.224) -> (-40325.557, -11824.224)
  line L739 (-32000, -5900) -> (-32000, -9700)
  line L740 (-32000, -9700) -> (-36447.7114, -9700)
  line L741 (-31900, -10500) -> (-31900, -13900)
  line L742 (-31900, -13900) -> (-36427.7515, -13900)
  line L743 (-36427.7515, -13900) -> (-36427.7515, -17506.808)
  line L744 (-32200, -10500) -> (-32200, -13600)
  line L745 (-32200, -13600) -> (-36727.7515, -13600)
  line L746 (-36727.7515, -13600) -> (-36727.7515, -17506.808)
  line L747 (-36447.7114, -9700) -> (-36447.7114, -13500)
  line L748 (-36447.7114, -13500) -> (-36447.7114, -13600)
  line L749 (-32200, -10500) -> (-31900, -10500)
  line L750 (-32300, -5900) -> (-32300, -9400)
  line L751 (-32300, -9400) -> (-36747.7114, -9400)
  line L752 (-36747.7114, -9400) -> (-36747.7114, -13500)
  line L753 (-36747.7114, -13500) -> (-36747.7114, -13600)
  line L754 (-36747.7114, -9400) -> (-36747.7114, -5300)
  line L755 (-36447.7114, -9400) -> (-36447.7114, -5300)
  line L756 (-32300, -5900) -> (-32000, -5900)
  line L757 (-36727.7515, -13600) -> (-36747.7114, -13600)
  line L758 (-36727.7515, -17506.808) -> (-36427.7515, -17506.808)
  line L759 (-36427.7515, -17506.808) -> (-32100, -17506.808)
  line L760 (-32100, -17506.808) -> (-32100, -15500)
  line L761 (-32100, -15500) -> (-31800, -15500)
  line L762 (-36427.7515, -17806.808) -> (-31800, -17806.808)
  line L763 (-31800, -17806.808) -> (-31800, -15800)
  line L764 (-31800, -15500) -> (-31800, -15800)
  line L765 (-31800, -17806.808) -> (-31800, -21841.7288)
  line L766 (-31800, -21841.7288) -> (-35200, -21841.7288)
  line L767 (-32100, -17806.808) -> (-32100, -21541.7288)
  line L768 (-32100, -21541.7288) -> (-35200, -21541.7288)
  line L769 (-35200, -21541.7288) -> (-35200, -21841.7288)
  line L770 (-36427.7515, -17806.808) -> (-36427.7515, -21700)
  line L771 (-36427.7515, -21700) -> (-36727.7515, -21700)
  line L772 (-36727.7515, -21700) -> (-36727.7515, -17800)
  line L773 (-36727.7515, -17800) -> (-40100, -17800)
  line L774 (-40100, -17800) -> (-40100, -21400)
  line L775 (-40100, -21400) -> (-37200, -21400)
  line L776 (-37200, -21400) -> (-37200, -21700)
  line L777 (-37200, -21700) -> (-40400, -21700)
  line L778 (-40400, -21700) -> (-40400, -13300)
  line L779 (-36727.7515, -17506.808) -> (-40100, -17506.808)
  line L780 (-40100, -17506.808) -> (-40100, -13300)
  line L781 (-40100, -13300) -> (-40400, -13300)
  line L782 (-37272.9626, -23397.9233) -> (-26452.1365, -23397.9233)
  line L783 (-26452.1365, -23397.9233) -> (-26452.1365, -30669.5185)
  line L784 (-37272.9626, -30669.5185) -> (-37272.9626, -23397.9233)
  line L785 (-28160.0906, -30369.5185) -> (-34121.938, -30369.5185)
  line L786 (-36972.9626, -30369.5185) -> (-36972.9626, -23697.9233)
  line L787 (-36972.9626, -23697.9233) -> (-26752.1365, -23697.9233)
  line L788 (-26752.1365, -23697.9233) -> (-26752.1365, -30369.5185)
  line L789 (-26752.1365, -27033.7209) -> (-36972.9626, -27033.7209)
  line L790 (-36972.9626, -27033.7209) -> (-36972.9626, -27333.7209)
  line L791 (-36972.9626, -27333.7209) -> (-26752.1365, -27333.7209)
  line L792 (-26752.1365, -27333.7209) -> (-26752.1365, -27033.7209)
  line L793 (-30988.2268, -27333.7209) -> (-31288.2268, -27333.7209)
  line L794 (-31288.2268, -27333.7209) -> (-31288.2268, -30369.5185)
  line L795 (-31288.2268, -30369.5185) -> (-30988.2268, -30369.5185)
  line L796 (-30988.2268, -30369.5185) -> (-30988.2268, -27333.7209)
  line L797 (-34121.938, -30369.5185) -> (-34121.938, -30669.5185)
  line L798 (-36972.9626, -30669.5185) -> (-36972.9626, -30369.5185)
  line L799 (-28160.0906, -30369.5185) -> (-28160.0906, -30669.5185)
  line L800 (-26752.1365, -30669.5185) -> (-26752.1365, -30369.5185)
  line L801 (-26452.1365, -30669.5185) -> (-26752.1365, -30669.5185)
  line L802 (-28160.0906, -30669.5185) -> (-34121.938, -30669.5185)
  line L803 (-36972.9626, -30669.5185) -> (-37272.9626, -30669.5185)
  line L804 (-5492.6505, -24449.2068) -> (-5492.6505, -30775.0235)
  line L805 (-24500, -30775.0235) -> (-24500, -23500)
  line L806 (-24200, -30475.0235) -> (-24200, -23800)
  line L807 (-5792.6505, -24449.2068) -> (-5792.6505, -30475.0235)
  line L808 (-23000, -23800) -> (-23000, -23500)
  line L809 (-24200, -23500) -> (-24200, -23800)
  line L810 (-15789.7616, -23800) -> (-15789.7616, -23500)
  line L811 (-16998.4164, -23500) -> (-16998.4164, -23800)
  line L812 (-9040.1308, -23500) -> (-9040.1308, -23800)
  line L813 (-9824.9716, -23800) -> (-9824.9716, -23500)
  line L814 (-5492.6505, -24449.2068) -> (-5792.6505, -24449.2068)
  line L815 (-5792.6505, -23800) -> (-5792.6505, -23500)
  line L816 (-8208.1996, -30475.0235) -> (-8208.1996, -30775.0235)
  line L817 (-5792.6505, -30775.0235) -> (-5792.6505, -30475.0235)
  line L818 (-16841.4482, -30475.0235) -> (-16841.4482, -30775.0235)
  line L819 (-14188.6864, -30775.0235) -> (-14188.6864, -30475.0235)
  line L820 (-22774.8445, -30475.0235) -> (-22774.8445, -30775.0235)
  line L821 (-24200, -30775.0235) -> (-24200, -30475.0235)
  line L822 (-24200, -30775.0235) -> (-24500, -30775.0235)
  line L823 (-23000, -23800) -> (-20153.4763, -23800)
  line L824 (-20153.4763, -23800) -> (-20153.4763, -27137.5117)
  line L825 (-20153.4763, -27137.5117) -> (-24200, -27137.5117)
  line L826 (-24200, -27137.5117) -> (-24200, -23800)
  line L827 (-19853.4763, -23500) -> (-19853.4763, -27437.5117)
  line L828 (-19853.4763, -27437.5117) -> (-24500, -27437.5117)
  line L829 (-24500, -27437.5117) -> (-24500, -23500)
  line L830 (-24500, -23500) -> (-24200, -23500)
  line L831 (-24500, -23500) -> (-24200, -23500)
  line L832 (-23000, -23500) -> (-19853.4763, -23500)
  line L833 (-19853.4763, -27437.5117) -> (-5792.6505, -27437.5117)
  line L834 (-19853.4763, -27137.5117) -> (-5792.6505, -27137.5117)
  line L835 (-23000, -23800) -> (-16998.4164, -23800)
  line L836 (-23000, -23500) -> (-16998.4164, -23500)
  line L837 (-15789.7616, -23500) -> (-9824.9716, -23500)
  line L838 (-9040.1308, -23500) -> (-5792.6505, -23500)
  line L839 (-15789.7616, -23800) -> (-9824.9716, -23800)
  line L840 (-9040.1308, -23800) -> (-5792.6505, -23800)
  line L841 (-9040.1308, -23800) -> (-8740.1308, -23800)
  line L842 (-8740.1308, -23800) -> (-8740.1308, -27137.5117)
  line L843 (-8740.1308, -27137.5117) -> (-9040.1308, -27137.5117)
  line L844 (-9040.1308, -27137.5117) -> (-9040.1308, -23800)
  line L845 (-13027.122, -23800) -> (-12727.122, -23800)
  line L846 (-12727.122, -23800) -> (-12727.122, -27137.5117)
  line L847 (-12727.122, -27137.5117) -> (-13027.122, -27137.5117)
  line L848 (-13027.122, -27137.5117) -> (-13027.122, -23800)
  line L849 (-19853.4763, -27437.5117) -> (-19553.4763, -27437.5117)
  line L850 (-19553.4763, -27437.5117) -> (-19553.4763, -30475.0235)
  line L851 (-19553.4763, -30475.0235) -> (-19853.4763, -30475.0235)
  line L852 (-19853.4763, -30475.0235) -> (-19853.4763, -27437.5117)
  line L853 (-11237.685, -27437.5117) -> (-10937.685, -27437.5117)
  line L854 (-10937.685, -27437.5117) -> (-10937.685, -30475.0235)
  line L855 (-10937.685, -30475.0235) -> (-11237.685, -30475.0235)
  line L856 (-11237.685, -30475.0235) -> (-11237.685, -27437.5117)
  line L857 (-16841.4482, -30775.0235) -> (-22774.8445, -30775.0235)
  line L858 (-8208.1996, -30475.0235) -> (-14188.6864, -30475.0235)
  line L859 (-16841.4482, -30475.0235) -> (-22774.8445, -30475.0235)
  line L860 (-5492.6505, -30775.0235) -> (-5792.6505, -30775.0235)
  line L861 (-8208.1996, -30775.0235) -> (-14188.6864, -30775.0235)
  line L862 (-30500, -2500) -> (-17733.768, -2500)
  line L863 (-17733.768, -21548.9807) -> (-30500, -21548.9807)
  line L864 (-18033.768, -21248.9807) -> (-30200, -21248.9807)
  line L865 (-30200, -2800) -> (-18033.768, -2800)
  line L866 (-25024.4191, -2800) -> (-23500, -2800)
  line L867 (-23500, -2800) -> (-23500, -10000)
  line L868 (-23500, -10000) -> (-25024.4191, -10000)
  line L869 (-25024.4191, -10000) -> (-25024.4191, -2800)
  line L870 (-25024.4191, -14817.1949) -> (-23500, -14817.1949)
  line L871 (-23500, -14817.1949) -> (-23500, -21248.9807)
  line L872 (-23500, -21248.9807) -> (-25024.4191, -21248.9807)
  line L873 (-25024.4191, -21248.9807) -> (-25024.4191, -14817.1949)
  line L874 (-25900, -9900) -> (-30200, -9900)
  line L875 (-30200, -9900) -> (-30200, -10200)
  line L876 (-30200, -10200) -> (-25900, -10200)
  line L877 (-25900, -10200) -> (-25900, -9900)
  line L878 (-22200, -9800) -> (-18033.768, -9800)
  line L879 (-18033.768, -9800) -> (-18033.768, -10100)
  line L880 (-18033.768, -10100) -> (-22200, -10100)
  line L881 (-22200, -10100) -> (-22200, -9800)
  line L882 (-30500, -12400) -> (-30200, -12400)
  line L883 (-30200, -13800) -> (-30500, -13800)
  line L884 (-18033.768, -10100) -> (-17733.768, -10100)
  line L885 (-17733.768, -14892.6106) -> (-18033.768, -14892.6106)
  line L886 (-30200, -21248.9807) -> (-30200, -13800)
  line L887 (-30200, -12400) -> (-30200, -2800)
  line L888 (-30500, -21548.9807) -> (-30500, -13800)
  line L889 (-30500, -12400) -> (-30500, -2500)
  line L890 (-17733.768, -2500) -> (-17733.768, -10100)
  line L891 (-17733.768, -14892.6106) -> (-17733.768, -21548.9807)
  line L892 (-18033.768, -2800) -> (-18033.768, -10100)
  line L893 (-18033.768, -14892.6106) -> (-18033.768, -21248.9807)
  line L894 (-18033.768, -14892.6106) -> (-22210.8504, -14892.6106)
  line L895 (-22210.8504, -14892.6106) -> (-22210.8504, -15192.6106)
  line L896 (-22210.8504, -15192.6106) -> (-18033.768, -15192.6106)
  line L897 (-18033.768, -15192.6106) -> (-18033.768, -14892.6106)
  line L898 (-26100, -14800) -> (-30200, -14800)
  line L899 (-30200, -14800) -> (-30200, -15100)
  line L900 (-30200, -15100) -> (-26100, -15100)
  line L901 (-26100, -15100) -> (-26100, -14800)
  line L902 (-14459.0053, -14770.8764) -> (-14459.0053, -21146.3937)
  line L903 (-14459.0053, -21146.3937) -> (-1100, -21146.3937)
  line L904 (-1100, -21146.3937) -> (-1100, -14900)
  line L905 (-1100, -14900) -> (-13200, -14900)
  line L906 (-14759.0053, -14770.8764) -> (-14759.0053, -21446.3937)
  line L907 (-14759.0053, -21446.3937) -> (-800, -21446.3937)
  line L908 (-800, -21446.3937) -> (-800, -14600)
  line L909 (-800, -14600) -> (-13200, -14600)
  line L910 (-13200, -14600) -> (-13200, -14900)
  line L911 (-14459.0053, -14770.8764) -> (-14759.0053, -14770.8764)
  line L912 (-800, -14600) -> (-1100, -14600)
  line L913 (-1100, -14600) -> (-1100, -13000)
  line L914 (-1100, -13000) -> (-800, -13000)
  line L915 (-800, -13000) -> (-800, -14600)
  line L916 (-904.3735, -11252.1545) -> (-904.3735, -2837.0745)